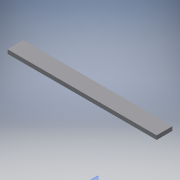
# Autodesk Inventor part: Wheel mount bottom
Saved by Autodesk Inventor 2018.2 (Build 222227000, 227)
## iProperties
Created: 2018-02-27
Part Number: Wheel mount bottom
Material: Generic
Document SubType Name: Modeling
Designer: owner
Density: 1 g/cm^3
Appearance: Default
Author: owner
Autodesk Inventor part; units mm, degrees
ref_plane "YZ Plane" through (0, 0, 0) normal (1, 0, 0) x (0, 1, 0)
ref_plane "XZ Plane" through (0, 0, 0) normal (0, 1, 0) x (-1, 0, 0)
ref_plane "XY Plane" through (0, 0, 0) normal (0, 0, 1) x (1, 0, 0)
sketch "Sketch1" plane through (0, 0, 0) normal (0, 0, 1) x (1, 0, 0)
  line L0 (-535.871, 526.142) -> (-535.871, 399.142) projected
  line L1 (-535.871, 399.142) -> (162.0194, 399.142) projected
  line L2 (162.0194, 526.142) -> (-535.871, 526.142) projected
  line L3 (-535.871, 399.142) -> (162.0194, 399.142)
  line L4 (162.0194, 399.142) -> (162.0194, 418.192)
  line L5 (162.0194, 418.192) -> (-535.871, 418.192)
  line L6 (-535.871, 418.192) -> (-535.871, 399.142)
  line L7 (162.0194, 399.142) -> (162.0194, 526.142) projected
  point P0 (0, 0)
  dimension "d0" = 19.05
  dimension "d1" = 697.8904
  constraints: 8 end point, 2 parallel, 1 horizontal, 1 perpendicular
  measures "d0" distance of L4.end L3.end
  measures "d1" distance of L4.end L5.end
extrude "Extrusion1" add sketch "Sketch1" along normal blind 76.2 contours L5 L4 L1 L0
body "Solid1"
